Autodesk Inventor part; units mm, degrees
(part 2 of 3)
  line L455 (76.25, 138.9015) -> (78.25, 136.9015) construction
  line L456 (78.75, 141.4015) -> (73.75, 136.4015)
  arc A259 (71.6287, 138.5228) -> (73.75, 136.4015) centre (72.6893, 137.4621) ccw
  line L457 (77.6893, 142.4621) -> (72.6893, 137.4621) construction
  line L458 (71.6287, 138.5228) -> (76.6287, 143.5228)
  arc A260 (78.75, 141.4015) -> (76.6287, 143.5228) centre (77.6893, 142.4621) ccw
  line L459 (84.3107, 145.3787) -> (79.3107, 150.3787) construction
  line L460 (78.25, 149.318) -> (83.25, 144.318)
  arc A261 (83.25, 144.318) -> (85.3713, 146.4393) centre (84.3107, 145.3787) ccw
  line L461 (85.3713, 146.4393) -> (80.3713, 151.4393)
  arc A262 (80.3713, 151.4393) -> (78.25, 149.318) centre (79.3107, 150.3787) ccw
  line L462 (76.25, 153.4393) -> (78.25, 151.4393) construction
  line L463 (78.75, 155.9393) -> (73.75, 150.9393)
  arc A263 (71.6287, 153.0607) -> (73.75, 150.9393) centre (72.6893, 152) ccw
  line L464 (77.6893, 157) -> (72.6893, 152) construction
  line L465 (71.6287, 153.0607) -> (76.6287, 158.0607)
  arc A264 (78.75, 155.9393) -> (76.6287, 158.0607) centre (77.6893, 157) ccw
  line L466 (69.7728, 0) -> (64.7728, 5) construction
  line L467 (63.7121, 3.9393) -> (68.7121, -1.0607)
  arc A265 (68.7121, -1.0607) -> (70.8335, 1.0607) centre (69.7728, 0) ccw
  line L468 (70.8335, 1.0607) -> (65.8335, 6.0607)
  arc A266 (65.8335, 6.0607) -> (63.7121, 3.9393) centre (64.7728, 5) ccw
  line L469 (61.7121, 8.0607) -> (63.7121, 6.0607) construction
  line L470 (64.2121, 10.5607) -> (59.2121, 5.5607)
  arc A267 (57.0908, 7.682) -> (59.2121, 5.5607) centre (58.1515, 6.6213) ccw
  line L471 (63.1515, 11.6213) -> (58.1515, 6.6213) construction
  line L472 (57.0908, 7.682) -> (62.0908, 12.682)
  arc A268 (64.2121, 10.5607) -> (62.0908, 12.682) centre (63.1515, 11.6213) ccw
  line L473 (69.7728, 14.5379) -> (64.7728, 19.5379) construction
  line L474 (63.7121, 18.4772) -> (68.7121, 13.4772)
  arc A269 (68.7121, 13.4772) -> (70.8335, 15.5985) centre (69.7728, 14.5379) ccw
  line L475 (70.8335, 15.5985) -> (65.8335, 20.5985)
  arc A270 (65.8335, 20.5985) -> (63.7121, 18.4772) centre (64.7728, 19.5379) ccw
  line L476 (61.7121, 22.5985) -> (63.7121, 20.5985) construction
  line L477 (64.2121, 25.0985) -> (59.2121, 20.0985)
  arc A271 (57.0908, 22.2198) -> (59.2121, 20.0985) centre (58.1515, 21.1592) ccw
  line L478 (63.1515, 26.1592) -> (58.1515, 21.1592) construction
  line L479 (57.0908, 22.2198) -> (62.0908, 27.2198)
  arc A272 (64.2121, 25.0985) -> (62.0908, 27.2198) centre (63.1515, 26.1592) ccw
  line L480 (69.7728, 29.0757) -> (64.7728, 34.0757) construction
  line L481 (63.7121, 33.0151) -> (68.7121, 28.0151)
  arc A273 (68.7121, 28.0151) -> (70.8335, 30.1364) centre (69.7728, 29.0757) ccw
  line L482 (70.8335, 30.1364) -> (65.8335, 35.1364)
  arc A274 (65.8335, 35.1364) -> (63.7121, 33.0151) centre (64.7728, 34.0757) ccw
  line L483 (61.7121, 37.1364) -> (63.7121, 35.1364) construction
  line L484 (64.2121, 39.6364) -> (59.2121, 34.6364)
  arc A275 (57.0908, 36.7577) -> (59.2121, 34.6364) centre (58.1515, 35.6971) ccw
  line L485 (63.1515, 40.6971) -> (58.1515, 35.6971) construction
  line L486 (57.0908, 36.7577) -> (62.0908, 41.7577)
  arc A276 (64.2121, 39.6364) -> (62.0908, 41.7577) centre (63.1515, 40.6971) ccw
  line L487 (69.7728, 43.6136) -> (64.7728, 48.6136) construction
  line L488 (63.7121, 47.5529) -> (68.7121, 42.5529)
  arc A277 (68.7121, 42.5529) -> (70.8335, 44.6743) centre (69.7728, 43.6136) ccw
  line L489 (70.8335, 44.6743) -> (65.8335, 49.6743)
  arc A278 (65.8335, 49.6743) -> (63.7121, 47.5529) centre (64.7728, 48.6136) ccw
  line L490 (61.7121, 51.6743) -> (63.7121, 49.6743) construction
  line L491 (64.2121, 54.1743) -> (59.2121, 49.1743)
  arc A279 (57.0908, 51.2956) -> (59.2121, 49.1743) centre (58.1515, 50.2349) ccw
  line L492 (63.1515, 55.2349) -> (58.1515, 50.2349) construction
  line L493 (57.0908, 51.2956) -> (62.0908, 56.2956)
  arc A280 (64.2121, 54.1743) -> (62.0908, 56.2956) centre (63.1515, 55.2349) ccw
  line L494 (69.7728, 58.1515) -> (64.7728, 63.1515) construction
  line L495 (63.7121, 62.0908) -> (68.7121, 57.0908)
  arc A281 (68.7121, 57.0908) -> (70.8335, 59.2121) centre (69.7728, 58.1515) ccw
  line L496 (70.8335, 59.2121) -> (65.8335, 64.2121)
  arc A282 (65.8335, 64.2121) -> (63.7121, 62.0908) centre (64.7728, 63.1515) ccw
  line L497 (61.7121, 66.2121) -> (63.7121, 64.2121) construction
  line L498 (64.2121, 68.7121) -> (59.2121, 63.7121)
  arc A283 (57.0908, 65.8335) -> (59.2121, 63.7121) centre (58.1515, 64.7728) ccw
  line L499 (63.1515, 69.7728) -> (58.1515, 64.7728) construction
  line L500 (57.0908, 65.8335) -> (62.0908, 70.8335)
  arc A284 (64.2121, 68.7121) -> (62.0908, 70.8335) centre (63.1515, 69.7728) ccw
  line L501 (69.7728, 72.6893) -> (64.7728, 77.6893) construction
  line L502 (63.7121, 76.6287) -> (68.7121, 71.6287)
  arc A285 (68.7121, 71.6287) -> (70.8335, 73.75) centre (69.7728, 72.6893) ccw
  line L503 (70.8335, 73.75) -> (65.8335, 78.75)
  arc A286 (65.8335, 78.75) -> (63.7121, 76.6287) centre (64.7728, 77.6893) ccw
  line L504 (61.7121, 80.75) -> (63.7121, 78.75) construction
  line L505 (64.2121, 83.25) -> (59.2121, 78.25)
  arc A287 (57.0908, 80.3713) -> (59.2121, 78.25) centre (58.1515, 79.3107) ccw
  line L506 (63.1515, 84.3107) -> (58.1515, 79.3107) construction
  line L507 (57.0908, 80.3713) -> (62.0908, 85.3713)
  arc A288 (64.2121, 83.25) -> (62.0908, 85.3713) centre (63.1515, 84.3107) ccw
  line L508 (69.7728, 87.2272) -> (64.7728, 92.2272) construction
  line L509 (63.7121, 91.1665) -> (68.7121, 86.1665)
  arc A289 (68.7121, 86.1665) -> (70.8335, 88.2879) centre (69.7728, 87.2272) ccw
  line L510 (70.8335, 88.2879) -> (65.8335, 93.2879)
  arc A290 (65.8335, 93.2879) -> (63.7121, 91.1665) centre (64.7728, 92.2272) ccw
  line L511 (61.7121, 95.2879) -> (63.7121, 93.2879) construction
  line L512 (64.2121, 97.7879) -> (59.2121, 92.7879)
  arc A291 (57.0908, 94.9092) -> (59.2121, 92.7879) centre (58.1515, 93.8485) ccw
  line L513 (63.1515, 98.8485) -> (58.1515, 93.8485) construction
  line L514 (57.0908, 94.9092) -> (62.0908, 99.9092)
  arc A292 (64.2121, 97.7879) -> (62.0908, 99.9092) centre (63.1515, 98.8485) ccw
  line L515 (69.7728, 101.7651) -> (64.7728, 106.7651) construction
  line L516 (63.7121, 105.7044) -> (68.7121, 100.7044)
  arc A293 (68.7121, 100.7044) -> (70.8335, 102.8257) centre (69.7728, 101.7651) ccw
  line L517 (70.8335, 102.8257) -> (65.8335, 107.8257)
  arc A294 (65.8335, 107.8257) -> (63.7121, 105.7044) centre (64.7728, 106.7651) ccw
  line L518 (61.7121, 109.8257) -> (63.7121, 107.8257) construction
  line L519 (64.2121, 112.3257) -> (59.2121, 107.3257)
  arc A295 (57.0908, 109.4471) -> (59.2121, 107.3257) centre (58.1515, 108.3864) ccw
  line L520 (63.1515, 113.3864) -> (58.1515, 108.3864) construction
  line L521 (57.0908, 109.4471) -> (62.0908, 114.4471)
  arc A296 (64.2121, 112.3257) -> (62.0908, 114.4471) centre (63.1515, 113.3864) ccw
  line L522 (69.7728, 116.3029) -> (64.7728, 121.3029) construction
  line L523 (63.7121, 120.2423) -> (68.7121, 115.2423)
  arc A297 (68.7121, 115.2423) -> (70.8335, 117.3636) centre (69.7728, 116.3029) ccw
  line L524 (70.8335, 117.3636) -> (65.8335, 122.3636)
  arc A298 (65.8335, 122.3636) -> (63.7121, 120.2423) centre (64.7728, 121.3029) ccw
  line L525 (61.7121, 124.3636) -> (63.7121, 122.3636) construction
  line L526 (64.2121, 126.8636) -> (59.2121, 121.8636)
  arc A299 (57.0908, 123.9849) -> (59.2121, 121.8636) centre (58.1515, 122.9243) ccw
  line L527 (63.1515, 127.9243) -> (58.1515, 122.9243) construction
  line L528 (57.0908, 123.9849) -> (62.0908, 128.9849)
  arc A300 (64.2121, 126.8636) -> (62.0908, 128.9849) centre (63.1515, 127.9243) ccw
  line L529 (69.7728, 130.8408) -> (64.7728, 135.8408) construction
  line L530 (63.7121, 134.7802) -> (68.7121, 129.7802)
  arc A301 (68.7121, 129.7802) -> (70.8335, 131.9015) centre (69.7728, 130.8408) ccw
  line L531 (70.8335, 131.9015) -> (65.8335, 136.9015)
  arc A302 (65.8335, 136.9015) -> (63.7121, 134.7802) centre (64.7728, 135.8408) ccw
  line L532 (61.7121, 138.9015) -> (63.7121, 136.9015) construction
  line L533 (64.2121, 141.4015) -> (59.2121, 136.4015)
  arc A303 (57.0908, 138.5228) -> (59.2121, 136.4015) centre (58.1515, 137.4621) ccw
  line L534 (63.1515, 142.4621) -> (58.1515, 137.4621) construction
  line L535 (57.0908, 138.5228) -> (62.0908, 143.5228)
  arc A304 (64.2121, 141.4015) -> (62.0908, 143.5228) centre (63.1515, 142.4621) ccw
  line L536 (69.7728, 145.3787) -> (64.7728, 150.3787) construction
  line L537 (63.7121, 149.318) -> (68.7121, 144.318)
  arc A305 (68.7121, 144.318) -> (70.8335, 146.4393) centre (69.7728, 145.3787) ccw
  line L538 (70.8335, 146.4393) -> (65.8335, 151.4393)
  arc A306 (65.8335, 151.4393) -> (63.7121, 149.318) centre (64.7728, 150.3787) ccw
  line L539 (61.7121, 153.4393) -> (63.7121, 151.4393) construction
  line L540 (64.2121, 155.9393) -> (59.2121, 150.9393)
  arc A307 (57.0908, 153.0607) -> (59.2121, 150.9393) centre (58.1515, 152) ccw
  line L541 (63.1515, 157) -> (58.1515, 152) construction
  line L542 (57.0908, 153.0607) -> (62.0908, 158.0607)
  arc A308 (64.2121, 155.9393) -> (62.0908, 158.0607) centre (63.1515, 157) ccw
  line L543 (55.2349, 0) -> (50.2349, 5) construction
  line L544 (49.1743, 3.9393) -> (54.1743, -1.0607)
  arc A309 (54.1743, -1.0607) -> (56.2956, 1.0607) centre (55.2349, 0) ccw
  line L545 (56.2956, 1.0607) -> (51.2956, 6.0607)
  arc A310 (51.2956, 6.0607) -> (49.1743, 3.9393) centre (50.2349, 5) ccw
  line L546 (47.1743, 8.0607) -> (49.1743, 6.0607) construction
  line L547 (49.6743, 10.5607) -> (44.6743, 5.5607)
  arc A311 (42.5529, 7.682) -> (44.6743, 5.5607) centre (43.6136, 6.6213) ccw
  line L548 (48.6136, 11.6213) -> (43.6136, 6.6213) construction
  line L549 (42.5529, 7.682) -> (47.5529, 12.682)
  arc A312 (49.6743, 10.5607) -> (47.5529, 12.682) centre (48.6136, 11.6213) ccw
  line L550 (55.2349, 14.5379) -> (50.2349, 19.5379) construction
  line L551 (49.1743, 18.4772) -> (54.1743, 13.4772)
  arc A313 (54.1743, 13.4772) -> (56.2956, 15.5985) centre (55.2349, 14.5379) ccw
  line L552 (56.2956, 15.5985) -> (51.2956, 20.5985)
  arc A314 (51.2956, 20.5985) -> (49.1743, 18.4772) centre (50.2349, 19.5379) ccw
  line L553 (47.1743, 22.5985) -> (49.1743, 20.5985) construction
  line L554 (49.6743, 25.0985) -> (44.6743, 20.0985)
  arc A315 (42.5529, 22.2198) -> (44.6743, 20.0985) centre (43.6136, 21.1592) ccw
  line L555 (48.6136, 26.1592) -> (43.6136, 21.1592) construction
  line L556 (42.5529, 22.2198) -> (47.5529, 27.2198)
  arc A316 (49.6743, 25.0985) -> (47.5529, 27.2198) centre (48.6136, 26.1592) ccw
  line L557 (55.2349, 29.0757) -> (50.2349, 34.0757) construction
  line L558 (49.1743, 33.0151) -> (54.1743, 28.0151)
  arc A317 (54.1743, 28.0151) -> (56.2956, 30.1364) centre (55.2349, 29.0757) ccw
  line L559 (56.2956, 30.1364) -> (51.2956, 35.1364)
  arc A318 (51.2956, 35.1364) -> (49.1743, 33.0151) centre (50.2349, 34.0757) ccw
  line L560 (47.1743, 37.1364) -> (49.1743, 35.1364) construction
  line L561 (49.6743, 39.6364) -> (44.6743, 34.6364)
  arc A319 (42.5529, 36.7577) -> (44.6743, 34.6364) centre (43.6136, 35.6971) ccw
  line L562 (48.6136, 40.6971) -> (43.6136, 35.6971) construction
  line L563 (42.5529, 36.7577) -> (47.5529, 41.7577)
  arc A320 (49.6743, 39.6364) -> (47.5529, 41.7577) centre (48.6136, 40.6971) ccw
  line L564 (55.2349, 43.6136) -> (50.2349, 48.6136) construction
  line L565 (49.1743, 47.5529) -> (54.1743, 42.5529)
  arc A321 (54.1743, 42.5529) -> (56.2956, 44.6743) centre (55.2349, 43.6136) ccw
  line L566 (56.2956, 44.6743) -> (51.2956, 49.6743)
  arc A322 (51.2956, 49.6743) -> (49.1743, 47.5529) centre (50.2349, 48.6136) ccw
  line L567 (47.1743, 51.6743) -> (49.1743, 49.6743) construction
  line L568 (49.6743, 54.1743) -> (44.6743, 49.1743)
  arc A323 (42.5529, 51.2956) -> (44.6743, 49.1743) centre (43.6136, 50.2349) ccw
  line L569 (48.6136, 55.2349) -> (43.6136, 50.2349) construction
  line L570 (42.5529, 51.2956) -> (47.5529, 56.2956)
  arc A324 (49.6743, 54.1743) -> (47.5529, 56.2956) centre (48.6136, 55.2349) ccw
  line L571 (55.2349, 58.1515) -> (50.2349, 63.1515) construction
  line L572 (49.1743, 62.0908) -> (54.1743, 57.0908)
  arc A325 (54.1743, 57.0908) -> (56.2956, 59.2121) centre (55.2349, 58.1515) ccw
  line L573 (56.2956, 59.2121) -> (51.2956, 64.2121)
  arc A326 (51.2956, 64.2121) -> (49.1743, 62.0908) centre (50.2349, 63.1515) ccw
  line L574 (47.1743, 66.2121) -> (49.1743, 64.2121) construction
  line L575 (49.6743, 68.7121) -> (44.6743, 63.7121)
  arc A327 (42.5529, 65.8335) -> (44.6743, 63.7121) centre (43.6136, 64.7728) ccw
  line L576 (48.6136, 69.7728) -> (43.6136, 64.7728) construction
  line L577 (42.5529, 65.8335) -> (47.5529, 70.8335)
  arc A328 (49.6743, 68.7121) -> (47.5529, 70.8335) centre (48.6136, 69.7728) ccw
  line L578 (55.2349, 72.6893) -> (50.2349, 77.6893) construction
  line L579 (49.1743, 76.6287) -> (54.1743, 71.6287)
  arc A329 (54.1743, 71.6287) -> (56.2956, 73.75) centre (55.2349, 72.6893) ccw
  line L580 (56.2956, 73.75) -> (51.2956, 78.75)
  arc A330 (51.2956, 78.75) -> (49.1743, 76.6287) centre (50.2349, 77.6893) ccw
  line L581 (47.1743, 80.75) -> (49.1743, 78.75) construction
  line L582 (49.6743, 83.25) -> (44.6743, 78.25)
  arc A331 (42.5529, 80.3713) -> (44.6743, 78.25) centre (43.6136, 79.3107) ccw
  line L583 (48.6136, 84.3107) -> (43.6136, 79.3107) construction
  line L584 (42.5529, 80.3713) -> (47.5529, 85.3713)
  arc A332 (49.6743, 83.25) -> (47.5529, 85.3713) centre (48.6136, 84.3107) ccw
  line L585 (55.2349, 87.2272) -> (50.2349, 92.2272) construction
  line L586 (49.1743, 91.1665) -> (54.1743, 86.1665)
  arc A333 (54.1743, 86.1665) -> (56.2956, 88.2879) centre (55.2349, 87.2272) ccw
  line L587 (56.2956, 88.2879) -> (51.2956, 93.2879)
  arc A334 (51.2956, 93.2879) -> (49.1743, 91.1665) centre (50.2349, 92.2272) ccw
  line L588 (47.1743, 95.2879) -> (49.1743, 93.2879) construction
  line L589 (49.6743, 97.7879) -> (44.6743, 92.7879)
  arc A335 (42.5529, 94.9092) -> (44.6743, 92.7879) centre (43.6136, 93.8485) ccw
  line L590 (48.6136, 98.8485) -> (43.6136, 93.8485) construction
  line L591 (42.5529, 94.9092) -> (47.5529, 99.9092)
  arc A336 (49.6743, 97.7879) -> (47.5529, 99.9092) centre (48.6136, 98.8485) ccw
  line L592 (55.2349, 101.7651) -> (50.2349, 106.7651) construction
  line L593 (49.1743, 105.7044) -> (54.1743, 100.7044)
  arc A337 (54.1743, 100.7044) -> (56.2956, 102.8257) centre (55.2349, 101.7651) ccw
  line L594 (56.2956, 102.8257) -> (51.2956, 107.8257)
  arc A338 (51.2956, 107.8257) -> (49.1743, 105.7044) centre (50.2349, 106.7651) ccw
  line L595 (47.1743, 109.8257) -> (49.1743, 107.8257) construction
  line L596 (49.6743, 112.3257) -> (44.6743, 107.3257)
  arc A339 (42.5529, 109.4471) -> (44.6743, 107.3257) centre (43.6136, 108.3864) ccw
  line L597 (48.6136, 113.3864) -> (43.6136, 108.3864) construction
  line L598 (42.5529, 109.4471) -> (47.5529, 114.4471)
  arc A340 (49.6743, 112.3257) -> (47.5529, 114.4471) centre (48.6136, 113.3864) ccw
  line L599 (55.2349, 116.3029) -> (50.2349, 121.3029) construction
  line L600 (49.1743, 120.2423) -> (54.1743, 115.2423)
  arc A341 (54.1743, 115.2423) -> (56.2956, 117.3636) centre (55.2349, 116.3029) ccw
  line L601 (56.2956, 117.3636) -> (51.2956, 122.3636)
  arc A342 (51.2956, 122.3636) -> (49.1743, 120.2423) centre (50.2349, 121.3029) ccw
  line L602 (47.1743, 124.3636) -> (49.1743, 122.3636) construction
  line L603 (49.6743, 126.8636) -> (44.6743, 121.8636)
  arc A343 (42.5529, 123.9849) -> (44.6743, 121.8636) centre (43.6136, 122.9243) ccw
  line L604 (48.6136, 127.9243) -> (43.6136, 122.9243) construction
  line L605 (42.5529, 123.9849) -> (47.5529, 128.9849)
  arc A344 (49.6743, 126.8636) -> (47.5529, 128.9849) centre (48.6136, 127.9243) ccw
  line L606 (55.2349, 130.8408) -> (50.2349, 135.8408) construction
  line L607 (49.1743, 134.7802) -> (54.1743, 129.7802)
  arc A345 (54.1743, 129.7802) -> (56.2956, 131.9015) centre (55.2349, 130.8408) ccw
  line L608 (56.2956, 131.9015) -> (51.2956, 136.9015)
  arc A346 (51.2956, 136.9015) -> (49.1743, 134.7802) centre (50.2349, 135.8408) ccw
  line L609 (47.1743, 138.9015) -> (49.1743, 136.9015) construction
  line L610 (49.6743, 141.4015) -> (44.6743, 136.4015)
  arc A347 (42.5529, 138.5228) -> (44.6743, 136.4015) centre (43.6136, 137.4621) ccw
  line L611 (48.6136, 142.4621) -> (43.6136, 137.4621) construction
  line L612 (42.5529, 138.5228) -> (47.5529, 143.5228)
  arc A348 (49.6743, 141.4015) -> (47.5529, 143.5228) centre (48.6136, 142.4621) ccw
  line L613 (55.2349, 145.3787) -> (50.2349, 150.3787) construction
  line L614 (49.1743, 149.318) -> (54.1743, 144.318)
  arc A349 (54.1743, 144.318) -> (56.2956, 146.4393) centre (55.2349, 145.3787) ccw
  line L615 (56.2956, 146.4393) -> (51.2956, 151.4393)
  arc A350 (51.2956, 151.4393) -> (49.1743, 149.318) centre (50.2349, 150.3787) ccw
  line L616 (47.1743, 153.4393) -> (49.1743, 151.4393) construction
  line L617 (49.6743, 155.9393) -> (44.6743, 150.9393)
  arc A351 (42.5529, 153.0607) -> (44.6743, 150.9393) centre (43.6136, 152) ccw
  line L618 (48.6136, 157) -> (43.6136, 152) construction
  line L619 (42.5529, 153.0607) -> (47.5529, 158.0607)
  arc A352 (49.6743, 155.9393) -> (47.5529, 158.0607) centre (48.6136, 157) ccw
  line L620 (40.6971, 0) -> (35.6971, 5) construction
  line L621 (34.6364, 3.9393) -> (39.6364, -1.0607)
  arc A353 (39.6364, -1.0607) -> (41.7577, 1.0607) centre (40.6971, 0) ccw
  line L622 (41.7577, 1.0607) -> (36.7577, 6.0607)
  arc A354 (36.7577, 6.0607) -> (34.6364, 3.9393) centre (35.6971, 5) ccw
  line L623 (32.6364, 8.0607) -> (34.6364, 6.0607) construction
  line L624 (35.1364, 10.5607) -> (30.1364, 5.5607)
  arc A355 (28.0151, 7.682) -> (30.1364, 5.5607) centre (29.0757, 6.6213) ccw
  line L625 (34.0757, 11.6213) -> (29.0757, 6.6213) construction
  line L626 (28.0151, 7.682) -> (33.0151, 12.682)
  arc A356 (35.1364, 10.5607) -> (33.0151, 12.682) centre (34.0757, 11.6213) ccw
  line L627 (40.6971, 14.5379) -> (35.6971, 19.5379) construction
  line L628 (34.6364, 18.4772) -> (39.6364, 13.4772)
  arc A357 (39.6364, 13.4772) -> (41.7577, 15.5985) centre (40.6971, 14.5379) ccw
  line L629 (41.7577, 15.5985) -> (36.7577, 20.5985)
  arc A358 (36.7577, 20.5985) -> (34.6364, 18.4772) centre (35.6971, 19.5379) ccw
  line L630 (32.6364, 22.5985) -> (34.6364, 20.5985) construction
  line L631 (35.1364, 25.0985) -> (30.1364, 20.0985)
  arc A359 (28.0151, 22.2198) -> (30.1364, 20.0985) centre (29.0757, 21.1592) ccw
  line L632 (34.0757, 26.1592) -> (29.0757, 21.1592) construction
  line L633 (28.0151, 22.2198) -> (33.0151, 27.2198)
  arc A360 (35.1364, 25.0985) -> (33.0151, 27.2198) centre (34.0757, 26.1592) ccw
  line L634 (40.6971, 29.0757) -> (35.6971, 34.0757) construction
  line L635 (34.6364, 33.0151) -> (39.6364, 28.0151)
  arc A361 (39.6364, 28.0151) -> (41.7577, 30.1364) centre (40.6971, 29.0757) ccw
  line L636 (41.7577, 30.1364) -> (36.7577, 35.1364)
  arc A362 (36.7577, 35.1364) -> (34.6364, 33.0151) centre (35.6971, 34.0757) ccw
  line L637 (32.6364, 37.1364) -> (34.6364, 35.1364) construction
  line L638 (35.1364, 39.6364) -> (30.1364, 34.6364)
  arc A363 (28.0151, 36.7577) -> (30.1364, 34.6364) centre (29.0757, 35.6971) ccw
  line L639 (34.0757, 40.6971) -> (29.0757, 35.6971) construction
  line L640 (28.0151, 36.7577) -> (33.0151, 41.7577)
  arc A364 (35.1364, 39.6364) -> (33.0151, 41.7577) centre (34.0757, 40.6971) ccw
  line L641 (40.6971, 43.6136) -> (35.6971, 48.6136) construction
  line L642 (34.6364, 47.5529) -> (39.6364, 42.5529)
  arc A365 (39.6364, 42.5529) -> (41.7577, 44.6743) centre (40.6971, 43.6136) ccw
  line L643 (41.7577, 44.6743) -> (36.7577, 49.6743)
  arc A366 (36.7577, 49.6743) -> (34.6364, 47.5529) centre (35.6971, 48.6136) ccw
  line L644 (32.6364, 51.6743) -> (34.6364, 49.6743) construction
  line L645 (35.1364, 54.1743) -> (30.1364, 49.1743)
  arc A367 (28.0151, 51.2956) -> (30.1364, 49.1743) centre (29.0757, 50.2349) ccw
  line L646 (34.0757, 55.2349) -> (29.0757, 50.2349) construction
  line L647 (28.0151, 51.2956) -> (33.0151, 56.2956)
  arc A368 (35.1364, 54.1743) -> (33.0151, 56.2956) centre (34.0757, 55.2349) ccw
  line L648 (40.6971, 58.1515) -> (35.6971, 63.1515) construction
  line L649 (34.6364, 62.0908) -> (39.6364, 57.0908)
  arc A369 (39.6364, 57.0908) -> (41.7577, 59.2121) centre (40.6971, 58.1515) ccw
  line L650 (41.7577, 59.2121) -> (36.7577, 64.2121)
  arc A370 (36.7577, 64.2121) -> (34.6364, 62.0908) centre (35.6971, 63.1515) ccw
  line L651 (32.6364, 66.2121) -> (34.6364, 64.2121) construction
  line L652 (35.1364, 68.7121) -> (30.1364, 63.7121)
  arc A371 (28.0151, 65.8335) -> (30.1364, 63.7121) centre (29.0757, 64.7728) ccw
  line L653 (34.0757, 69.7728) -> (29.0757, 64.7728) construction
  line L654 (28.0151, 65.8335) -> (33.0151, 70.8335)
  arc A372 (35.1364, 68.7121) -> (33.0151, 70.8335) centre (34.0757, 69.7728) ccw
  line L655 (40.6971, 72.6893) -> (35.6971, 77.6893) construction
  line L656 (34.6364, 76.6287) -> (39.6364, 71.6287)
  arc A373 (39.6364, 71.6287) -> (41.7577, 73.75) centre (40.6971, 72.6893) ccw
  line L657 (41.7577, 73.75) -> (36.7577, 78.75)
  arc A374 (36.7577, 78.75) -> (34.6364, 76.6287) centre (35.6971, 77.6893) ccw
  line L658 (32.6364, 80.75) -> (34.6364, 78.75) construction
  line L659 (35.1364, 83.25) -> (30.1364, 78.25)
  arc A375 (28.0151, 80.3713) -> (30.1364, 78.25) centre (29.0757, 79.3107) ccw
  line L660 (34.0757, 84.3107) -> (29.0757, 79.3107) construction
  line L661 (28.0151, 80.3713) -> (33.0151, 85.3713)
  arc A376 (35.1364, 83.25) -> (33.0151, 85.3713) centre (34.0757, 84.3107) ccw
  line L662 (40.6971, 87.2272) -> (35.6971, 92.2272) construction
  line L663 (34.6364, 91.1665) -> (39.6364, 86.1665)
  arc A377 (39.6364, 86.1665) -> (41.7577, 88.2879) centre (40.6971, 87.2272) ccw
  line L664 (41.7577, 88.2879) -> (36.7577, 93.2879)
  arc A378 (36.7577, 93.2879) -> (34.6364, 91.1665) centre (35.6971, 92.2272) ccw
  line L665 (32.6364, 95.2879) -> (34.6364, 93.2879) construction
  line L666 (35.1364, 97.7879) -> (30.1364, 92.7879)
  arc A379 (28.0151, 94.9092) -> (30.1364, 92.7879) centre (29.0757, 93.8485) ccw
  line L667 (34.0757, 98.8485) -> (29.0757, 93.8485) construction
  line L668 (28.0151, 94.9092) -> (33.0151, 99.9092)
  arc A380 (35.1364, 97.7879) -> (33.0151, 99.9092) centre (34.0757, 98.8485) ccw
  line L669 (40.6971, 101.7651) -> (35.6971, 106.7651) construction
  line L670 (34.6364, 105.7044) -> (39.6364, 100.7044)
  arc A381 (39.6364, 100.7044) -> (41.7577, 102.8257) centre (40.6971, 101.7651) ccw
  line L671 (41.7577, 102.8257) -> (36.7577, 107.8257)
  arc A382 (36.7577, 107.8257) -> (34.6364, 105.7044) centre (35.6971, 106.7651) ccw
  line L672 (32.6364, 109.8257) -> (34.6364, 107.8257) construction
  line L673 (35.1364, 112.3257) -> (30.1364, 107.3257)
  arc A383 (28.0151, 109.4471) -> (30.1364, 107.3257) centre (29.0757, 108.3864) ccw
  line L674 (34.0757, 113.3864) -> (29.0757, 108.3864) construction
  line L675 (28.0151, 109.4471) -> (33.0151, 114.4471)
  arc A384 (35.1364, 112.3257) -> (33.0151, 114.4471) centre (34.0757, 113.3864) ccw
  line L676 (40.6971, 116.3029) -> (35.6971, 121.3029) construction
  line L677 (34.6364, 120.2423) -> (39.6364, 115.2423)
  arc A385 (39.6364, 115.2423) -> (41.7577, 117.3636) centre (40.6971, 116.3029) ccw
  line L678 (41.7577, 117.3636) -> (36.7577, 122.3636)
  arc A386 (36.7577, 122.3636) -> (34.6364, 120.2423) centre (35.6971, 121.3029) ccw
  line L679 (32.6364, 124.3636) -> (34.6364, 122.3636) construction
  line L680 (35.1364, 126.8636) -> (30.1364, 121.8636)
  arc A387 (28.0151, 123.9849) -> (30.1364, 121.8636) centre (29.0757, 122.9243) ccw
  line L681 (34.0757, 127.9243) -> (29.0757, 122.9243) construction
  line L682 (28.0151, 123.9849) -> (33.0151, 128.9849)
  arc A388 (35.1364, 126.8636) -> (33.0151, 128.9849) centre (34.0757, 127.9243) ccw
  line L683 (40.6971, 130.8408) -> (35.6971, 135.8408) construction
  line L684 (34.6364, 134.7802) -> (39.6364, 129.7802)
  arc A389 (39.6364, 129.7802) -> (41.7577, 131.9015) centre (40.6971, 130.8408) ccw
  line L685 (41.7577, 131.9015) -> (36.7577, 136.9015)
  arc A390 (36.7577, 136.9015) -> (34.6364, 134.7802) centre (35.6971, 135.8408) ccw
  line L686 (32.6364, 138.9015) -> (34.6364, 136.9015) construction
  line L687 (35.1364, 141.4015) -> (30.1364, 136.4015)
  arc A391 (28.0151, 138.5228) -> (30.1364, 136.4015) centre (29.0757, 137.4621) ccw
  line L688 (34.0757, 142.4621) -> (29.0757, 137.4621) construction
  line L689 (28.0151, 138.5228) -> (33.0151, 143.5228)
  arc A392 (35.1364, 141.4015) -> (33.0151, 143.5228) centre (34.0757, 142.4621) ccw
  line L690 (40.6971, 145.3787) -> (35.6971, 150.3787) construction
  line L691 (34.6364, 149.318) -> (39.6364, 144.318)
  arc A393 (39.6364, 144.318) -> (41.7577, 146.4393) centre (40.6971, 145.3787) ccw
  line L692 (41.7577, 146.4393) -> (36.7577, 151.4393)
  arc A394 (36.7577, 151.4393) -> (34.6364, 149.318) centre (35.6971, 150.3787) ccw
  line L693 (32.6364, 153.4393) -> (34.6364, 151.4393) construction
  line L694 (35.1364, 155.9393) -> (30.1364, 150.9393)
  arc A395 (28.0151, 153.0607) -> (30.1364, 150.9393) centre (29.0757, 152) ccw
  line L695 (34.0757, 157) -> (29.0757, 152) construction
  line L696 (28.0151, 153.0607) -> (33.0151, 158.0607)
  arc A396 (35.1364, 155.9393) -> (33.0151, 158.0607) centre (34.0757, 157) ccw
  line L697 (26.1592, 0) -> (21.1592, 5) construction
  line L698 (20.0985, 3.9393) -> (25.0985, -1.0607)
  arc A397 (25.0985, -1.0607) -> (27.2198, 1.0607) centre (26.1592, 0) ccw
  line L699 (27.2198, 1.0607) -> (22.2198, 6.0607)
  arc A398 (22.2198, 6.0607) -> (20.0985, 3.9393) centre (21.1592, 5) ccw
  line L700 (18.0985, 8.0607) -> (20.0985, 6.0607) construction
  line L701 (20.5985, 10.5607) -> (15.5985, 5.5607)
  arc A399 (13.4772, 7.682) -> (15.5985, 5.5607) centre (14.5379, 6.6213) ccw
  line L702 (19.5379, 11.6213) -> (14.5379, 6.6213) construction
  line L703 (13.4772, 7.682) -> (18.4772, 12.682)
  arc A400 (20.5985, 10.5607) -> (18.4772, 12.682) centre (19.5379, 11.6213) ccw
  line L704 (26.1592, 14.5379) -> (21.1592, 19.5379) construction
  line L705 (20.0985, 18.4772) -> (25.0985, 13.4772)
  arc A401 (25.0985, 13.4772) -> (27.2198, 15.5985) centre (26.1592, 14.5379) ccw
  line L706 (27.2198, 15.5985) -> (22.2198, 20.5985)
  arc A402 (22.2198, 20.5985) -> (20.0985, 18.4772) centre (21.1592, 19.5379) ccw
  line L707 (18.0985, 22.5985) -> (20.0985, 20.5985) construction
  line L708 (20.5985, 25.0985) -> (15.5985, 20.0985)
  arc A403 (13.4772, 22.2198) -> (15.5985, 20.0985) centre (14.5379, 21.1592) ccw
  line L709 (19.5379, 26.1592) -> (14.5379, 21.1592) construction
  line L710 (13.4772, 22.2198) -> (18.4772, 27.2198)
  arc A404 (20.5985, 25.0985) -> (18.4772, 27.2198) centre (19.5379, 26.1592) ccw
  line L711 (26.1592, 29.0757) -> (21.1592, 34.0757) construction
  line L712 (20.0985, 33.0151) -> (25.0985, 28.0151)
  arc A405 (25.0985, 28.0151) -> (27.2198, 30.1364) centre (26.1592, 29.0757) ccw
  line L713 (27.2198, 30.1364) -> (22.2198, 35.1364)
  arc A406 (22.2198, 35.1364) -> (20.0985, 33.0151) centre (21.1592, 34.0757) ccw
  line L714 (18.0985, 37.1364) -> (20.0985, 35.1364) construction
  line L715 (20.5985, 39.6364) -> (15.5985, 34.6364)
  arc A407 (13.4772, 36.7577) -> (15.5985, 34.6364) centre (14.5379, 35.6971) ccw
  line L716 (19.5379, 40.6971) -> (14.5379, 35.6971) construction
  line L717 (13.4772, 36.7577) -> (18.4772, 41.7577)
  arc A408 (20.5985, 39.6364) -> (18.4772, 41.7577) centre (19.5379, 40.6971) ccw
  line L718 (26.1592, 43.6136) -> (21.1592, 48.6136) construction
  line L719 (20.0985, 47.5529) -> (25.0985, 42.5529)
  arc A409 (25.0985, 42.5529) -> (27.2198, 44.6743) centre (26.1592, 43.6136) ccw
  line L720 (27.2198, 44.6743) -> (22.2198, 49.6743)
  arc A410 (22.2198, 49.6743) -> (20.0985, 47.5529) centre (21.1592, 48.6136) ccw
  line L721 (18.0985, 51.6743) -> (20.0985, 49.6743) construction
  line L722 (20.5985, 54.1743) -> (15.5985, 49.1743)
  arc A411 (13.4772, 51.2956) -> (15.5985, 49.1743) centre (14.5379, 50.2349) ccw
  line L723 (19.5379, 55.2349) -> (14.5379, 50.2349) construction
  line L724 (13.4772, 51.2956) -> (18.4772, 56.2956)
  arc A412 (20.5985, 54.1743) -> (18.4772, 56.2956) centre (19.5379, 55.2349) ccw
  line L725 (26.1592, 58.1515) -> (21.1592, 63.1515) construction
  line L726 (20.0985, 62.0908) -> (25.0985, 57.0908)
  arc A413 (25.0985, 57.0908) -> (27.2198, 59.2121) centre (26.1592, 58.1515) ccw
  line L727 (27.2198, 59.2121) -> (22.2198, 64.2121)
  arc A414 (22.2198, 64.2121) -> (20.0985, 62.0908) centre (21.1592, 63.1515) ccw
  line L728 (18.0985, 66.2121) -> (20.0985, 64.2121) construction
  line L729 (20.5985, 68.7121) -> (15.5985, 63.7121)
  arc A415 (13.4772, 65.8335) -> (15.5985, 63.7121) centre (14.5379, 64.7728) ccw
  line L730 (19.5379, 69.7728) -> (14.5379, 64.7728) construction
  line L731 (13.4772, 65.8335) -> (18.4772, 70.8335)
  arc A416 (20.5985, 68.7121) -> (18.4772, 70.8335) centre (19.5379, 69.7728) ccw
  line L732 (26.1592, 72.6893) -> (21.1592, 77.6893) construction
  line L733 (20.0985, 76.6287) -> (25.0985, 71.6287)
  arc A417 (25.0985, 71.6287) -> (27.2198, 73.75) centre (26.1592, 72.6893) ccw
  line L734 (27.2198, 73.75) -> (22.2198, 78.75)
  arc A418 (22.2198, 78.75) -> (20.0985, 76.6287) centre (21.1592, 77.6893) ccw
  line L735 (18.0985, 80.75) -> (20.0985, 78.75) construction
  line L736 (20.5985, 83.25) -> (15.5985, 78.25)
  arc A419 (13.4772, 80.3713) -> (15.5985, 78.25) centre (14.5379, 79.3107) ccw
  line L737 (19.5379, 84.3107) -> (14.5379, 79.3107) construction
  line L738 (13.4772, 80.3713) -> (18.4772, 85.3713)
  arc A420 (20.5985, 83.25) -> (18.4772, 85.3713) centre (19.5379, 84.3107) ccw
  line L739 (26.1592, 87.2272) -> (21.1592, 92.2272) construction
  line L740 (20.0985, 91.1665) -> (25.0985, 86.1665)
  arc A421 (25.0985, 86.1665) -> (27.2198, 88.2879) centre (26.1592, 87.2272) ccw
  line L741 (27.2198, 88.2879) -> (22.2198, 93.2879)
  arc A422 (22.2198, 93.2879) -> (20.0985, 91.1665) centre (21.1592, 92.2272) ccw
  line L742 (18.0985, 95.2879) -> (20.0985, 93.2879) construction
  line L743 (20.5985, 97.7879) -> (15.5985, 92.7879)
  arc A423 (13.4772, 94.9092) -> (15.5985, 92.7879) centre (14.5379, 93.8485) ccw
  line L744 (19.5379, 98.8485) -> (14.5379, 93.8485) construction
  line L745 (13.4772, 94.9092) -> (18.4772, 99.9092)
  arc A424 (20.5985, 97.7879) -> (18.4772, 99.9092) centre (19.5379, 98.8485) ccw
  line L746 (26.1592, 101.7651) -> (21.1592, 106.7651) construction
  line L747 (20.0985, 105.7044) -> (25.0985, 100.7044)
  arc A425 (25.0985, 100.7044) -> (27.2198, 102.8257) centre (26.1592, 101.7651) ccw
  line L748 (27.2198, 102.8257) -> (22.2198, 107.8257)
  arc A426 (22.2198, 107.8257) -> (20.0985, 105.7044) centre (21.1592, 106.7651) ccw
  line L749 (18.0985, 109.8257) -> (20.0985, 107.8257) construction
  line L750 (20.5985, 112.3257) -> (15.5985, 107.3257)
  arc A427 (13.4772, 109.4471) -> (15.5985, 107.3257) centre (14.5379, 108.3864) ccw
  line L751 (19.5379, 113.3864) -> (14.5379, 108.3864) construction
  line L752 (13.4772, 109.4471) -> (18.4772, 114.4471)
  arc A428 (20.5985, 112.3257) -> (18.4772, 114.4471) centre (19.5379, 113.3864) ccw
  line L753 (26.1592, 116.3029) -> (21.1592, 121.3029) construction
  line L754 (20.0985, 120.2423) -> (25.0985, 115.2423)
  arc A429 (25.0985, 115.2423) -> (27.2198, 117.3636) centre (26.1592, 116.3029) ccw
  line L755 (27.2198, 117.3636) -> (22.2198, 122.3636)
  arc A430 (22.2198, 122.3636) -> (20.0985, 120.2423) centre (21.1592, 121.3029) ccw
  line L756 (18.0985, 124.3636) -> (20.0985, 122.3636) construction
  line L757 (20.5985, 126.8636) -> (15.5985, 121.8636)
  arc A431 (13.4772, 123.9849) -> (15.5985, 121.8636) centre (14.5379, 122.9243) ccw
  line L758 (19.5379, 127.9243) -> (14.5379, 122.9243) construction
  line L759 (13.4772, 123.9849) -> (18.4772, 128.9849)
  arc A432 (20.5985, 126.8636) -> (18.4772, 128.9849) centre (19.5379, 127.9243) ccw
  line L760 (26.1592, 130.8408) -> (21.1592, 135.8408) construction
  line L761 (20.0985, 134.7802) -> (25.0985, 129.7802)
  arc A433 (25.0985, 129.7802) -> (27.2198, 131.9015) centre (26.1592, 130.8408) ccw
  line L762 (27.2198, 131.9015) -> (22.2198, 136.9015)
  arc A434 (22.2198, 136.9015) -> (20.0985, 134.7802) centre (21.1592, 135.8408) ccw
  line L763 (18.0985, 138.9015) -> (20.0985, 136.9015) construction
  line L764 (20.5985, 141.4015) -> (15.5985, 136.4015)
  arc A435 (13.4772, 138.5228) -> (15.5985, 136.4015) centre (14.5379, 137.4621) ccw
  line L765 (19.5379, 142.4621) -> (14.5379, 137.4621) construction
  line L766 (13.4772, 138.5228) -> (18.4772, 143.5228)
  arc A436 (20.5985, 141.4015) -> (18.4772, 143.5228) centre (19.5379, 142.4621) ccw
  line L767 (26.1592, 145.3787) -> (21.1592, 150.3787) construction
  line L768 (20.0985, 149.318) -> (25.0985, 144.318)
  arc A437 (25.0985, 144.318) -> (27.2198, 146.4393) centre (26.1592, 145.3787) ccw
  line L769 (27.2198, 146.4393) -> (22.2198, 151.4393)
  arc A438 (22.2198, 151.4393) -> (20.0985, 149.318) centre (21.1592, 150.3787) ccw
  line L770 (18.0985, 153.4393) -> (20.0985, 151.4393) construction
  line L771 (20.5985, 155.9393) -> (15.5985, 150.9393)
  arc A439 (13.4772, 153.0607) -> (15.5985, 150.9393) centre (14.5379, 152) ccw
  line L772 (19.5379, 157) -> (14.5379, 152) construction
  line L773 (13.4772, 153.0607) -> (18.4772, 158.0607)
  arc A440 (20.5985, 155.9393) -> (18.4772, 158.0607) centre (19.5379, 157) ccw
  line L774 (11.6213, 0) -> (6.6213, 5) construction
  line L775 (5.5607, 3.9393) -> (10.5607, -1.0607)
  arc A441 (10.5607, -1.0607) -> (12.682, 1.0607) centre (11.6213, 0) ccw
  line L776 (12.682, 1.0607) -> (7.682, 6.0607)
  arc A442 (7.682, 6.0607) -> (5.5607, 3.9393) centre (6.6213, 5) ccw
  line L777 (3.5607, 8.0607) -> (5.5607, 6.0607) construction
  line L778 (6.0607, 10.5607) -> (1.0607, 5.5607)
  arc A443 (-1.0607, 7.682) -> (1.0607, 5.5607) centre (0, 6.6213) ccw
  line L779 (5, 11.6213) -> (0, 6.6213) construction
  line L780 (-1.0607, 7.682) -> (3.9393, 12.682)
  arc A444 (6.0607, 10.5607) -> (3.9393, 12.682) centre (5, 11.6213) ccw
  line L781 (11.6213, 14.5379) -> (6.6213, 19.5379) construction
  line L782 (5.5607, 18.4772) -> (10.5607, 13.4772)
  arc A445 (10.5607, 13.4772) -> (12.682, 15.5985) centre (11.6213, 14.5379) ccw
  line L783 (12.682, 15.5985) -> (7.682, 20.5985)
  arc A446 (7.682, 20.5985) -> (5.5607, 18.4772) centre (6.6213, 19.5379) ccw
  line L784 (3.5607, 22.5985) -> (5.5607, 20.5985) construction
  line L785 (6.0607, 25.0985) -> (1.0607, 20.0985)
  arc A447 (-1.0607, 22.2198) -> (1.0607, 20.0985) centre (0, 21.1592) ccw
  line L786 (5, 26.1592) -> (0, 21.1592) construction
  line L787 (-1.0607, 22.2198) -> (3.9393, 27.2198)
  arc A448 (6.0607, 25.0985) -> (3.9393, 27.2198) centre (5, 26.1592) ccw
  line L788 (11.6213, 29.0757) -> (6.6213, 34.0757) construction
  line L789 (5.5607, 33.0151) -> (10.5607, 28.0151)
  arc A449 (10.5607, 28.0151) -> (12.682, 30.1364) centre (11.6213, 29.0757) ccw
  line L790 (12.682, 30.1364) -> (7.682, 35.1364)
  arc A450 (7.682, 35.1364) -> (5.5607, 33.0151) centre (6.6213, 34.0757) ccw
  line L791 (3.5607, 37.1364) -> (5.5607, 35.1364) construction
  line L792 (6.0607, 39.6364) -> (1.0607, 34.6364)
  arc A451 (-1.0607, 36.7577) -> (1.0607, 34.6364) centre (0, 35.6971) ccw
  line L793 (5, 40.6971) -> (0, 35.6971) construction
  line L794 (-1.0607, 36.7577) -> (3.9393, 41.7577)
  arc A452 (6.0607, 39.6364) -> (3.9393, 41.7577) centre (5, 40.6971) ccw
  line L795 (11.6213, 43.6136) -> (6.6213, 48.6136) construction
  line L796 (5.5607, 47.5529) -> (10.5607, 42.5529)
  arc A453 (10.5607, 42.5529) -> (12.682, 44.6743) centre (11.6213, 43.6136) ccw
  line L797 (12.682, 44.6743) -> (7.682, 49.6743)
  arc A454 (7.682, 49.6743) -> (5.5607, 47.5529) centre (6.6213, 48.6136) ccw
  line L798 (3.5607, 51.6743) -> (5.5607, 49.6743) construction
  line L799 (6.0607, 54.1743) -> (1.0607, 49.1743)
  arc A455 (-1.0607, 51.2956) -> (1.0607, 49.1743) centre (0, 50.2349) ccw
  line L800 (5, 55.2349) -> (0, 50.2349) construction
  line L801 (-1.0607, 51.2956) -> (3.9393, 56.2956)
  arc A456 (6.0607, 54.1743) -> (3.9393, 56.2956) centre (5, 55.2349) ccw
  line L802 (11.6213, 58.1515) -> (6.6213, 63.1515) construction
  line L803 (5.5607, 62.0908) -> (10.5607, 57.0908)
  arc A457 (10.5607, 57.0908) -> (12.682, 59.2121) centre (11.6213, 58.1515) ccw
  line L804 (12.682, 59.2121) -> (7.682, 64.2121)
  arc A458 (7.682, 64.2121) -> (5.5607, 62.0908) centre (6.6213, 63.1515) ccw
  line L805 (3.5607, 66.2121) -> (5.5607, 64.2121) construction
  line L806 (6.0607, 68.7121) -> (1.0607, 63.7121)
  arc A459 (-1.0607, 65.8335) -> (1.0607, 63.7121) centre (0, 64.7728) ccw
  line L807 (5, 69.7728) -> (0, 64.7728) construction
  line L808 (-1.0607, 65.8335) -> (3.9393, 70.8335)
  arc A460 (6.0607, 68.7121) -> (3.9393, 70.8335) centre (5, 69.7728) ccw
  line L809 (11.6213, 72.6893) -> (6.6213, 77.6893) construction
  line L810 (5.5607, 76.6287) -> (10.5607, 71.6287)
  arc A461 (10.5607, 71.6287) -> (12.682, 73.75) centre (11.6213, 72.6893) ccw
  line L811 (12.682, 73.75) -> (7.682, 78.75)
  arc A462 (7.682, 78.75) -> (5.5607, 76.6287) centre (6.6213, 77.6893) ccw
  line L812 (3.5607, 80.75) -> (5.5607, 78.75) construction
  line L813 (6.0607, 83.25) -> (1.0607, 78.25)
  arc A463 (-1.0607, 80.3713) -> (1.0607, 78.25) centre (0, 79.3107) ccw
  line L814 (5, 84.3107) -> (0, 79.3107) construction
  line L815 (-1.0607, 80.3713) -> (3.9393, 85.3713)
  arc A464 (6.0607, 83.25) -> (3.9393, 85.3713) centre (5, 84.3107) ccw
  line L816 (11.6213, 87.2272) -> (6.6213, 92.2272) construction
  line L817 (5.5607, 91.1665) -> (10.5607, 86.1665)
  arc A465 (10.5607, 86.1665) -> (12.682, 88.2879) centre (11.6213, 87.2272) ccw
  line L818 (12.682, 88.2879) -> (7.682, 93.2879)
  arc A466 (7.682, 93.2879) -> (5.5607, 91.1665) centre (6.6213, 92.2272) ccw
  line L819 (3.5607, 95.2879) -> (5.5607, 93.2879) construction
  line L820 (6.0607, 97.7879) -> (1.0607, 92.7879)
  arc A467 (-1.0607, 94.9092) -> (1.0607, 92.7879) centre (0, 93.8485) ccw
  line L821 (5, 98.8485) -> (0, 93.8485) construction
  line L822 (-1.0607, 94.9092) -> (3.9393, 99.9092)
  arc A468 (6.0607, 97.7879) -> (3.9393, 99.9092) centre (5, 98.8485) ccw
  line L823 (11.6213, 101.7651) -> (6.6213, 106.7651) construction
  line L824 (5.5607, 105.7044) -> (10.5607, 100.7044)
  arc A469 (10.5607, 100.7044) -> (12.682, 102.8257) centre (11.6213, 101.7651) ccw
  line L825 (12.682, 102.8257) -> (7.682, 107.8257)
  arc A470 (7.682, 107.8257) -> (5.5607, 105.7044) centre (6.6213, 106.7651) ccw
  line L826 (3.5607, 109.8257) -> (5.5607, 107.8257) construction
  line L827 (6.0607, 112.3257) -> (1.0607, 107.3257)
  arc A471 (-1.0607, 109.4471) -> (1.0607, 107.3257) centre (0, 108.3864) ccw
  line L828 (5, 113.3864) -> (0, 108.3864) construction
  line L829 (-1.0607, 109.4471) -> (3.9393, 114.4471)
  arc A472 (6.0607, 112.3257) -> (3.9393, 114.4471) centre (5, 113.3864) ccw
  line L830 (11.6213, 116.3029) -> (6.6213, 121.3029) construction
  line L831 (5.5607, 120.2423) -> (10.5607, 115.2423)
  arc A473 (10.5607, 115.2423) -> (12.682, 117.3636) centre (11.6213, 116.3029) ccw
  line L832 (12.682, 117.3636) -> (7.682, 122.3636)
  arc A474 (7.682, 122.3636) -> (5.5607, 120.2423) centre (6.6213, 121.3029) ccw
  line L833 (3.5607, 124.3636) -> (5.5607, 122.3636) construction
  line L834 (6.0607, 126.8636) -> (1.0607, 121.8636)
  arc A475 (-1.0607, 123.9849) -> (1.0607, 121.8636) centre (0, 122.9243) ccw
  line L835 (5, 127.9243) -> (0, 122.9243) construction
  line L836 (-1.0607, 123.9849) -> (3.9393, 128.9849)
  arc A476 (6.0607, 126.8636) -> (3.9393, 128.9849) centre (5, 127.9243) ccw
  line L837 (11.6213, 130.8408) -> (6.6213, 135.8408) construction
  line L838 (5.5607, 134.7802) -> (10.5607, 129.7802)
  arc A477 (10.5607, 129.7802) -> (12.682, 131.9015) centre (11.6213, 130.8408) ccw
  line L839 (12.682, 131.9015) -> (7.682, 136.9015)
  arc A478 (7.682, 136.9015) -> (5.5607, 134.7802) centre (6.6213, 135.8408) ccw
  line L840 (3.5607, 138.9015) -> (5.5607, 136.9015) construction
  line L841 (6.0607, 141.4015) -> (1.0607, 136.4015)
  arc A479 (-1.0607, 138.5228) -> (1.0607, 136.4015) centre (0, 137.4621) ccw
  line L842 (5, 142.4621) -> (0, 137.4621) construction
  line L843 (-1.0607, 138.5228) -> (3.9393, 143.5228)
  arc A480 (6.0607, 141.4015) -> (3.9393, 143.5228) centre (5, 142.4621) ccw
  line L844 (11.6213, 145.3787) -> (6.6213, 150.3787) construction
  line L845 (5.5607, 149.318) -> (10.5607, 144.318)
  arc A481 (10.5607, 144.318) -> (12.682, 146.4393) centre (11.6213, 145.3787) ccw
  line L846 (12.682, 146.4393) -> (7.682, 151.4393)
  arc A482 (7.682, 151.4393) -> (5.5607, 149.318) centre (6.6213, 150.3787) ccw
  line L847 (3.5607, 153.4393) -> (5.5607, 151.4393) construction
  line L848 (6.0607, 155.9393) -> (1.0607, 150.9393)
  arc A483 (-1.0607, 153.0607) -> (1.0607, 150.9393) centre (0, 152) ccw
  line L849 (5, 157) -> (0, 152) construction
  line L850 (-1.0607, 153.0607) -> (3.9393, 158.0607)
  arc A484 (6.0607, 155.9393) -> (3.9393, 158.0607) centre (5, 157) ccw
  point P0 (154.5, 2.5)
  point P1 (147.8787, 9.1213)
  point P2 (0, 171.5379)
  point P3 (147.8787, 23.6592)
  point P4 (154.5, 17.0379)
  point P5 (0, 186.0757)
  point P6 (147.8787, 38.1971)
  point P7 (154.5, 31.5757)
  point P8 (0, 200.6136)
  point P9 (147.8787, 52.7349)
  point P10 (154.5, 46.1136)
  point P11 (0, 215.1515)
  point P12 (147.8787, 67.2728)
  point P13 (154.5, 60.6515)
  point P14 (0, 229.6893)
  point P15 (147.8787, 81.8107)
  point P16 (154.5, 75.1893)
  point P17 (0, 244.2272)
  point P18 (147.8787, 96.3485)
  point P19 (154.5, 89.7272)
  point P20 (0, 258.7651)
  point P21 (147.8787, 110.8864)
  point P22 (154.5, 104.2651)
  point P23 (0, 273.3029)
  point P24 (147.8787, 125.4243)
  point P25 (154.5, 118.8029)
  point P26 (0, 287.8408)
  point P27 (147.8787, 139.9621)
  point P28 (154.5, 133.3408)
  point P29 (0, 302.3787)
  point P30 (147.8787, 154.5)
  point P31 (154.5, 147.8787)
  point P32 (-14.5379, 157)
  point P33 (133.3408, 9.1213)
  point P34 (139.9621, 2.5)
  point P35 (-14.5379, 171.5379)
  point P36 (133.3408, 23.6592)
  point P37 (139.9621, 17.0379)
  point P38 (-14.5379, 186.0757)
  point P39 (133.3408, 38.1971)
  point P40 (139.9621, 31.5757)
  point P41 (-14.5379, 200.6136)
  point P42 (133.3408, 52.7349)
  point P43 (139.9621, 46.1136)
  point P44 (-14.5379, 215.1515)
  point P45 (133.3408, 67.2728)
  point P46 (139.9621, 60.6515)
  point P47 (-14.5379, 229.6893)
  point P48 (133.3408, 81.8107)
  point P49 (139.9621, 75.1893)
  point P50 (-14.5379, 244.2272)
  point P51 (133.3408, 96.3485)
  point P52 (139.9621, 89.7272)
  point P53 (-14.5379, 258.7651)
  point P54 (133.3408, 110.8864)
  point P55 (139.9621, 104.2651)
  point P56 (-14.5379, 273.3029)
  point P57 (133.3408, 125.4243)
  point P58 (139.9621, 118.8029)
  point P59 (-14.5379, 287.8408)
  point P60 (133.3408, 139.9621)
  point P61 (139.9621, 133.3408)
  point P62 (-14.5379, 302.3787)
  point P63 (133.3408, 154.5)
  point P64 (139.9621, 147.8787)
  point P65 (-29.0757, 157)
  point P66 (118.8029, 9.1213)
  point P67 (125.4243, 2.5)
  point P68 (-29.0757, 171.5379)
  point P69 (118.8029, 23.6592)
  point P70 (125.4243, 17.0379)
  point P71 (-29.0757, 186.0757)
  point P72 (118.8029, 38.1971)
  point P73 (125.4243, 31.5757)
  point P74 (-29.0757, 200.6136)
  point P75 (118.8029, 52.7349)
  point P76 (125.4243, 46.1136)
  point P77 (-29.0757, 215.1515)
  point P78 (118.8029, 67.2728)
  point P79 (125.4243, 60.6515)
  point P80 (-29.0757, 229.6893)
  point P81 (118.8029, 81.8107)
  point P82 (125.4243, 75.1893)
  point P83 (-29.0757, 244.2272)
  point P84 (118.8029, 96.3485)
  point P85 (125.4243, 89.7272)
  point P86 (-29.0757, 258.7651)
  point P87 (118.8029, 110.8864)
  point P88 (125.4243, 104.2651)
  point P89 (-29.0757, 273.3029)
  point P90 (118.8029, 125.4243)
  point P91 (125.4243, 118.8029)
  point P92 (-29.0757, 287.8408)
  point P93 (118.8029, 139.9621)
  point P94 (125.4243, 133.3408)
  point P95 (-29.0757, 302.3787)
  point P96 (118.8029, 154.5)
  point P97 (125.4243, 147.8787)
  point P98 (-43.6136, 157)
  point P99 (104.2651, 9.1213)
  point P100 (110.8864, 2.5)
  point P101 (-43.6136, 171.5379)
  point P102 (104.2651, 23.6592)
  point P103 (110.8864, 17.0379)
  point P104 (-43.6136, 186.0757)
  point P105 (104.2651, 38.1971)
  point P106 (110.8864, 31.5757)
  point P107 (-43.6136, 200.6136)
  point P108 (104.2651, 52.7349)
  point P109 (110.8864, 46.1136)
  point P110 (-43.6136, 215.1515)
  point P111 (104.2651, 67.2728)
  point P112 (110.8864, 60.6515)
  point P113 (-43.6136, 229.6893)
  point P114 (104.2651, 81.8107)
  point P115 (110.8864, 75.1893)
  point P116 (-43.6136, 244.2272)
  point P117 (104.2651, 96.3485)
  point P118 (110.8864, 89.7272)
  point P119 (-43.6136, 258.7651)
  point P120 (104.2651, 110.8864)
  point P121 (110.8864, 104.2651)
  point P122 (-43.6136, 273.3029)
  point P123 (104.2651, 125.4243)
  point P124 (110.8864, 118.8029)
  point P125 (-43.6136, 287.8408)
  point P126 (104.2651, 139.9621)
  point P127 (110.8864, 133.3408)
  point P128 (-43.6136, 302.3787)
  point P129 (104.2651, 154.5)
  point P130 (110.8864, 147.8787)
  point P131 (-58.1515, 157)
  point P132 (89.7272, 9.1213)
  point P133 (96.3485, 2.5)
  point P134 (-58.1515, 171.5379)
  point P135 (89.7272, 23.6592)
  point P136 (96.3485, 17.0379)
  point P137 (-58.1515, 186.0757)
  point P138 (89.7272, 38.1971)
  point P139 (96.3485, 31.5757)
  point P140 (-58.1515, 200.6136)
  point P141 (89.7272, 52.7349)
  point P142 (96.3485, 46.1136)
  point P143 (-58.1515, 215.1515)
  point P144 (89.7272, 67.2728)
  point P145 (96.3485, 60.6515)
  point P146 (-58.1515, 229.6893)
  point P147 (89.7272, 81.8107)
  point P148 (96.3485, 75.1893)
  point P149 (-58.1515, 244.2272)
  point P150 (89.7272, 96.3485)
  point P151 (96.3485, 89.7272)
  point P152 (-58.1515, 258.7651)
  point P153 (89.7272, 110.8864)
  point P154 (96.3485, 104.2651)
  point P155 (-58.1515, 273.3029)
  point P156 (89.7272, 125.4243)
  point P157 (96.3485, 118.8029)
  point P158 (-58.1515, 287.8408)
  point P159 (89.7272, 139.9621)
  point P160 (96.3485, 133.3408)
  point P161 (-58.1515, 302.3787)
  point P162 (89.7272, 154.5)
  point P163 (96.3485, 147.8787)
  point P164 (-72.6893, 157)
  point P165 (75.1893, 9.1213)
  point P166 (81.8107, 2.5)
  point P167 (-72.6893, 171.5379)
  point P168 (75.1893, 23.6592)
  point P169 (81.8107, 17.0379)
  point P170 (-72.6893, 186.0757)
  point P171 (75.1893, 38.1971)
  point P172 (81.8107, 31.5757)
  point P173 (-72.6893, 200.6136)
  point P174 (75.1893, 52.7349)
  point P175 (81.8107, 46.1136)
  point P176 (-72.6893, 215.1515)
  point P177 (75.1893, 67.2728)
  point P178 (81.8107, 60.6515)
  point P179 (-72.6893, 229.6893)
  point P180 (75.1893, 81.8107)
  point P181 (81.8107, 75.1893)
  point P182 (-72.6893, 244.2272)
  point P183 (75.1893, 96.3485)
  point P184 (81.8107, 89.7272)
  point P185 (-72.6893, 258.7651)
  point P186 (75.1893, 110.8864)
  point P187 (81.8107, 104.2651)
  point P188 (-72.6893, 273.3029)
  point P189 (75.1893, 125.4243)
  point P190 (81.8107, 118.8029)
  point P191 (-72.6893, 287.8408)
  point P192 (75.1893, 139.9621)
  point P193 (81.8107, 133.3408)
  point P194 (-72.6893, 302.3787)
  point P195 (75.1893, 154.5)
  point P196 (81.8107, 147.8787)
  point P197 (-87.2272, 157)
  point P198 (60.6515, 9.1213)
  point P199 (67.2728, 2.5)
  dimension "d101" = 5
  dimension "d102" = 1.5
  dimension "d103" = 2
  dimension "d106" = 14.5379
  dimension "d109" = 14.5379
  constraints: 2186 end point, 969 point on circle, 484 centre point, 244 point on line, 8 tangent, 4 parallel, 3 midpoint, 3 perpendicular, 2 horizontal, 1 equal radius, 1 vertical, 3360 other
  measures "d101" horizontal distance of L0.end L4.end
  measures "d102" radius of A2
  measures "d103" horizontal distance of L10.start L10.end
  measures "d106" distance of L0.end L11.start
  measures "d109" distance of L0.end L81.start